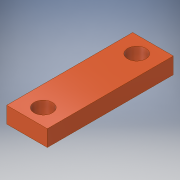
# Autodesk Inventor part: Spreader Belt clamp
Saved by Autodesk Inventor 2018 (Build 220112000, 112)
## iProperties
Created: 2013-10-16
Part Number: Spreader Belt clamp
Material: ABS Plastic
Document SubType Name: Modeling
Designer: Gabriel Smolnycki
Mass: 1.17953 g
Surface Area: 9.9748 cm^2
Volume: 1.11277 cm^3
Density: 1.06 g/cm^3
Appearance: Smooth - Light Orange
Author: Gabriel Smolnycki
Sending System: SolidWorks 2017
Last Author: Gabriel Smolnycki
Last Saved: 2017-09-14
Autodesk Inventor part; units mm, degrees
ref_plane "YZ Plane" through (0, 0, 0) normal (1, 0, 0) x (0, 1, 0)
ref_plane "XZ Plane" through (0, 0, 0) normal (0, 1, 0) x (-1, 0, 0)
ref_plane "Work Plane1" through (0, 0, 15.5) normal (0, 0, 1) x (1, 0, 0)
sketch "Sketch1" plane through (0, 0, 15.5) normal (0, 0, 1) x (1, 0, 0)
  line L0 (5, 4) -> (5, 0)
  line L1 (-5, 4) -> (5, 4)
  line L2 (-5, 0) -> (5, 0)
  line L3 (-5, 4) -> (-5, 0)
  constraints: 8 end point, 2 horizontal, 2 vertical
extrude "Extrusion1" add sketch "Sketch1" against normal blind 31
hole "Hole2" at (0, 4, -11.5) direction (0, -1, 0) diameter 4.5 depth 4
sketch "Sketch2" plane through (-5, 4, 15.5) normal (0, 1, 0) x (1, 0, 0)
  point P0 (5, 27)
hole "Hole1" at (0, 4, 11.5) direction (0, -1, 0) diameter 4.5 depth 4
sketch "Sketch3" plane through (-5, 4, 15.5) normal (0, 1, 0) x (1, 0, 0)
  point P0 (5, 4)
body "Solid3"
